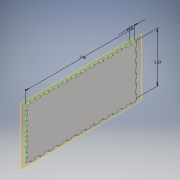
# Autodesk Inventor part: caja_lateral
Saved by Autodesk Inventor 2019 (Build 230136000, 136)
## iProperties
Created: 2018-05-30
Part Number: caja_lateral
Material: Generic
Document SubType Name: Modeling
Designer: seba
Density: 1 g/cm^3
Appearance: Default
Author: seba
Autodesk Inventor part; units mm, degrees
ref_plane "YZ Plane" through (0, 0, 0) normal (1, 0, 0) x (0, 1, 0)
ref_plane "XZ Plane" through (0, 0, 0) normal (0, 1, 0) x (-1, 0, 0)
ref_plane "XY Plane" through (0, 0, 0) normal (0, 0, 1) x (1, 0, 0)
sketch "Sketch1" plane through (0, 0, 0) normal (1, 0, 0) x (0, 1, 0)
  line L0 (-15.3344, -12.7912) -> (-12.3344, -12.7912)
  line L1 (-12.3344, -12.7912) -> (-12.3344, -22.7912)
  line L2 (-12.3344, -22.7912) -> (-15.3344, -22.7912)
  line L3 (-15.3344, -22.7912) -> (-15.3344, -32.7912)
  line L4 (-15.3344, -32.7912) -> (-12.3344, -32.7912)
  line L5 (-12.3344, -32.7912) -> (-12.3344, -42.7912)
  line L6 (-12.3344, -42.7912) -> (-15.3344, -42.7912)
  line L7 (-15.3344, -42.7912) -> (-15.3344, -52.7912)
  line L8 (-15.3344, -52.7912) -> (-12.3344, -52.7912)
  line L9 (-12.3344, -52.7912) -> (-12.3344, -62.7912)
  line L10 (-12.3344, -62.7912) -> (-15.3344, -62.7912)
  line L11 (-15.3344, -62.7912) -> (-15.3344, -72.7912)
  line L12 (-15.3344, -72.7912) -> (-12.3344, -72.7912)
  line L13 (-12.3344, -72.7912) -> (-12.3344, -82.7912)
  line L14 (-12.3344, -82.7912) -> (-15.3344, -82.7912)
  line L15 (-15.3344, -82.7912) -> (-15.3344, -92.7912)
  line L16 (-15.3344, -92.7912) -> (-12.3344, -92.7912)
  line L17 (-12.3344, -92.7912) -> (-12.3344, -102.7912)
  line L18 (-12.3344, -102.7912) -> (-15.3344, -102.7912)
  line L19 (-15.3344, -102.7912) -> (-15.3344, -112.7912)
  line L20 (-15.3344, -112.7912) -> (-12.3344, -112.7912)
  line L21 (-12.3344, -112.7912) -> (-12.3344, -122.7912)
  line L22 (-12.3344, -122.7912) -> (-15.3344, -122.7912)
  line L23 (-12.3344, -122.7912) -> (-15.3344, -122.7912)
  line L24 (-12.3344, -122.7912) -> (-15.3344, -122.7912)
  line L25 (-15.3344, -122.7912) -> (-15.3344, -132.7912)
  line L26 (-15.3344, -132.7912) -> (-12.3344, -132.7912)
  line L27 (-12.3344, -132.7912) -> (-12.3344, -142.7912)
  line L28 (-12.3344, -142.7912) -> (-15.3344, -142.7912)
  line L29 (-15.3344, -142.7912) -> (-15.3344, -152.7912)
  line L30 (-15.3344, -152.7912) -> (-12.3344, -152.7912)
  line L31 (-12.3344, -152.7912) -> (-12.3344, -162.7912)
  line L32 (-12.3344, -162.7912) -> (-15.3344, -162.7912)
  line L33 (-15.3344, -162.7912) -> (-15.3344, -172.7912)
  line L34 (-15.3344, -172.7912) -> (-12.3344, -172.7912)
  line L35 (-12.3344, -172.7912) -> (-12.3344, -182.7912)
  line L36 (-12.3344, -182.7912) -> (-15.3344, -182.7912)
  line L37 (-15.3344, -182.7912) -> (-15.3344, -192.7912)
  line L38 (-15.3344, -192.7912) -> (-12.3344, -192.7912)
  line L39 (-12.3344, -192.7912) -> (-12.3344, -202.7912)
  line L40 (-12.3344, -202.7912) -> (-15.3344, -202.7912)
  line L41 (-15.3344, -202.7912) -> (-15.3344, -212.7912)
  line L42 (-15.3344, -212.7912) -> (-12.3344, -212.7912)
  line L43 (-12.3344, -212.7912) -> (-12.3344, -222.7912)
  line L44 (-12.3344, -222.7912) -> (-15.3344, -222.7912)
  line L45 (-15.3344, -222.7912) -> (-15.3344, -232.7912)
  line L46 (-15.3344, -232.7912) -> (-12.3344, -232.7912)
  line L47 (-12.3344, -232.7912) -> (-12.3344, -242.7912)
  line L48 (-12.3344, -242.7912) -> (-15.3344, -242.7912)
  line L49 (-15.3344, -12.7912) -> (-15.3344, -2.7912)
  line L50 (-15.3344, -242.7912) -> (-15.3344, -245.7912)
  line L51 (-15.3344, -245.7912) -> (-25.3344, -245.7912)
  line L52 (-25.3344, -245.7912) -> (-25.3344, -242.7912)
  line L53 (-25.3344, -242.7912) -> (-35.3344, -242.7912)
  line L54 (-35.3344, -242.7912) -> (-35.3344, -245.7912)
  line L55 (-35.3344, -245.7912) -> (-45.3344, -245.7912)
  line L56 (-45.3344, -245.7912) -> (-45.3344, -242.7912)
  line L57 (-45.3344, -242.7912) -> (-55.3344, -242.7912)
  line L58 (-55.3344, -242.7912) -> (-55.3344, -245.7912)
  line L59 (-55.3344, -245.7912) -> (-65.3344, -245.7912)
  line L60 (-65.3344, -245.7912) -> (-65.3344, -242.7912)
  line L61 (-65.3344, -242.7912) -> (-75.3344, -242.7912)
  line L62 (-75.3344, -242.7912) -> (-75.3344, -245.7912)
  line L63 (-75.3344, -245.7912) -> (-85.3344, -245.7912)
  line L64 (-85.3344, -245.7912) -> (-85.3344, -242.7912)
  line L65 (-85.3344, -242.7912) -> (-95.3344, -242.7912)
  line L66 (-95.3344, -242.7912) -> (-95.3344, -245.7912)
  line L67 (-95.3344, -245.7912) -> (-105.3344, -245.7912)
  line L68 (-105.3344, -245.7912) -> (-105.3344, -242.7912)
  line L69 (-105.3344, -242.7912) -> (-115.3344, -242.7912)
  line L70 (-115.3344, -242.7912) -> (-115.3344, -245.7912)
  line L71 (-115.3344, -245.7912) -> (-125.3344, -245.7912)
  line L72 (-125.3344, -245.7912) -> (-125.3344, -242.7912)
  line L73 (-125.3344, -242.7912) -> (-128.3344, -242.7912)
  line L74 (-128.3344, -242.7912) -> (-128.3344, -232.7912)
  line L75 (-128.3344, -232.7912) -> (-125.3344, -232.7912)
  line L76 (-125.3344, -232.7912) -> (-125.3344, -222.7912)
  line L77 (-125.3344, -222.7912) -> (-128.3344, -222.7912)
  line L78 (-128.3344, -222.7912) -> (-128.3344, -212.7912)
  line L79 (-128.3344, -212.7912) -> (-125.3344, -212.7912)
  line L80 (-125.3344, -212.7912) -> (-125.3344, -202.7912)
  line L81 (-125.3344, -202.7912) -> (-128.3344, -202.7912)
  line L82 (-128.3344, -202.7912) -> (-128.3344, -192.7912)
  line L83 (-128.3344, -192.7912) -> (-125.3344, -192.7912)
  line L84 (-125.3344, -192.7912) -> (-125.3344, -182.7912)
  line L85 (-125.3344, -182.7912) -> (-128.3344, -182.7912)
  line L86 (-128.3344, -182.7912) -> (-128.3344, -172.7912)
  line L87 (-128.3344, -172.7912) -> (-125.3344, -172.7912)
  line L88 (-125.3344, -172.7912) -> (-125.3344, -162.7912)
  line L89 (-125.3344, -162.7912) -> (-128.3344, -162.7912)
  line L90 (-128.3344, -162.7912) -> (-128.3344, -152.7912)
  line L91 (-128.3344, -152.7912) -> (-125.3344, -152.7912)
  line L92 (-125.3344, -152.7912) -> (-125.3344, -142.7912)
  line L93 (-125.3344, -142.7912) -> (-128.3344, -142.7912)
  line L94 (-128.3344, -142.7912) -> (-128.3344, -132.7912)
  line L95 (-128.3344, -132.7912) -> (-125.3344, -132.7912)
  line L96 (-125.3344, -132.7912) -> (-125.3344, -122.7912)
  line L97 (-125.3344, -122.7912) -> (-128.3344, -122.7912)
  line L98 (-128.3344, -122.7912) -> (-128.3344, -112.7912)
  line L99 (-128.3344, -112.7912) -> (-125.3344, -112.7912)
  line L100 (-125.3344, -112.7912) -> (-125.3344, -102.7912)
  line L101 (-125.3344, -102.7912) -> (-128.3344, -102.7912)
  line L102 (-128.3344, -102.7912) -> (-128.3344, -92.7912)
  line L103 (-128.3344, -92.7912) -> (-125.3344, -92.7912)
  line L104 (-125.3344, -92.7912) -> (-125.3344, -82.7912)
  line L105 (-125.3344, -82.7912) -> (-128.3344, -82.7912)
  line L106 (-128.3344, -82.7912) -> (-128.3344, -72.7912)
  line L107 (-128.3344, -72.7912) -> (-125.3344, -72.7912)
  line L108 (-125.3344, -72.7912) -> (-125.3344, -62.7912)
  line L109 (-125.3344, -62.7912) -> (-128.3344, -62.7912)
  line L110 (-128.3344, -62.7912) -> (-128.3344, -52.7912)
  line L111 (-128.3344, -52.7912) -> (-125.3344, -52.7912)
  line L112 (-125.3344, -52.7912) -> (-125.3344, -42.7912)
  line L113 (-125.3344, -42.7912) -> (-128.3344, -42.7912)
  line L114 (-128.3344, -42.7912) -> (-128.3344, -32.7912)
  line L115 (-128.3344, -32.7912) -> (-125.3344, -32.7912)
  line L116 (-125.3344, -32.7912) -> (-125.3344, -22.7912)
  line L117 (-125.3344, -22.7912) -> (-128.3344, -22.7912)
  line L118 (-128.3344, -22.7912) -> (-128.3344, -12.7912)
  line L119 (-128.3344, -12.7912) -> (-125.3344, -12.7912)
  line L120 (-125.3344, -12.7912) -> (-125.3344, -2.7912)
  line L121 (-125.3344, -2.7912) -> (-115.3344, -2.7912)
  line L122 (-115.3344, -2.7912) -> (-115.3344, -5.7912)
  line L123 (-115.3344, -5.7912) -> (-105.3344, -5.7912)
  line L124 (-105.3344, -5.7912) -> (-105.3344, -2.7912)
  line L125 (-105.3344, -2.7912) -> (-95.3344, -2.7912)
  line L126 (-95.3344, -2.7912) -> (-95.3344, -5.7912)
  line L127 (-95.3344, -5.7912) -> (-85.3344, -5.7912)
  line L128 (-85.3344, -5.7912) -> (-85.3344, -2.7912)
  line L129 (-85.3344, -2.7912) -> (-75.3344, -2.7912)
  line L130 (-75.3344, -2.7912) -> (-75.3344, -5.7912)
  line L131 (-75.3344, -5.7912) -> (-65.3344, -5.7912)
  line L132 (-65.3344, -5.7912) -> (-65.3344, -2.7912)
  line L133 (-65.3344, -2.7912) -> (-55.3344, -2.7912)
  line L134 (-55.3344, -2.7912) -> (-55.3344, -5.7912)
  line L135 (-55.3344, -5.7912) -> (-45.3344, -5.7912)
  line L136 (-45.3344, -5.7912) -> (-45.3344, -2.7912)
  line L137 (-45.3344, -2.7912) -> (-35.3344, -2.7912)
  line L138 (-35.3344, -2.7912) -> (-35.3344, -5.7912)
  line L139 (-35.3344, -5.7912) -> (-25.3344, -5.7912)
  line L140 (-25.3344, -5.7912) -> (-25.3344, -2.7912)
  line L141 (-25.3344, -2.7912) -> (-15.3344, -2.7912)
  dimension "d91" = 240
  dimension "d92" = 110
  dimension "d93" = 10
  constraints: 284 end point, 102 point on line, 78 perpendicular, 6 horizontal, 6 vertical, 2 collinear
  measures "d91" vertical distance of L47.end L49.end
  measures "d92" distance of L71.end L50.end
  measures "d93" distance of L46.end L47.end
extrude "Extrusion1" add sketch "Sketch1" along normal blind 3
ref_plane "Work Plane1" through (1.5, 0, 0) normal (1, 0, 0) x (0, 0, -1)
body "Solid1"
